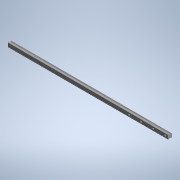
# Autodesk Inventor part: HSR30A128020 Rail(3.5)
Saved by Autodesk Inventor 2022 (Build 260153000, 153)
## iProperties
Category: PARTsolutions
Company: THK
Part Number: HSR30A128020 Rail(3.5)
Material: Generic
Catalog Web Link: www.cadenas.de
Description: Flange Type - Heavy Load HSR-A Rail-
Vendor: THK
Document SubType Name: Modeling
Designer: partserver
Manufacturer: THK
Mass: 162.345 g
Surface Area: 356.21 cm^2
Volume: 162.345 cm^3
Density: 1 g/cm^3
Appearance: PSOLRGB-192-192-192
PSOL_IDENT_0: {$CADENAS_DATA\23d-libs\thk\linear_motion_systems\lm_guide\lm_guide\lm_guide_hsr\four_taped_hole_typ
PSOL_IDENT_1: e\hsr_a\hsr_a_rail.prj},218 {VTYP=3D},{NB=HSR30A128020 Rail},{LINA=HSR30A128020 Rail},{NN=Flange Typ
PSOL_IDENT_2: e - Heavy Load HSR-A Rail},{DATE=08.06.2021 00:57:44},{GEOMDATE=24.12.2019 02:38:17},{VERSION=},{LIN
PSOL_IDENT_3: EID=60},{WBVAR=L,G,GX,TAPH},{WBNUMERIC=L,GX}  {NB=HSR30A128020 Rail},{LINA=HSR30A128020 Rail},{KT=DU
PSOL_IDENT_4: MMY},{MN=HSR30A},{NOB=1},{L=280.0},{G=},{GG='', 'Symmetrical (G1=G2)', 'A', 'Asymmetrical'},{GX=20},
PSOL_IDENT_5: {TAPH=},{GX1=20},{LMIN=98},{LEND=8640.00},{LMING=8.00},{LMAXG=32.00},{W1=28.00},{M1=26.00},{F=80.00}
PSOL_IDENT_6: ,{D1=9.00},{D2=14.00},{HM=12.00},{MAXL=3000.00},{GMIN=8},{GMX=20},{GMAX1=3.3},{G1=20},{G2=20},{NX=1}
PSOL_IDENT_7: ,{H3=7.00},{A=4},{LF=-20},{LM=320},{LL=620},{AA=3},{GMAX=32},{P=4},{PX=0},{VG=3},{VGG=20},{VG1=-1},{
PSOL_IDENT_8: VG2=4},{ND=4.000},{LT=2880},{GA=20.000},{X=0.000},{S1=8.000},{L1=15.000},{NOTE=MIN}
NB: HSR30A128020 Rail
NN: Flange Type - Heavy Load HSR-A Rail
NBSYN: $MN.$NOB.$L.$G.$GX.$TAPH. Rail
LINA: HSR30A128020 Rail
CATALOG: THK
MN: HSR30A
NOB: 1
L: 280
G: Symmetrical (G1=G2)
GX: 20
TAPH: Standard
LEND: 8640
LMING: 8
LMAXG: 32
W1: 28
M1: 26
F: 80
D1: 9
D2: 14
HM: 12
MAXL: 3000
H3: 7
ND: 4
GA: 20
X: 0
S1: 8
L1: 15
NOTE: 0
SUPPLIER: THK
ARTICLENO: HSR30A128020 Rail
BOMINFO: HSR30A128020 Rail
CREATOR: CADENAS GmbH
Title: HSR30A128020 Rail
Author: Cadenas PARTsolutions
Autodesk Inventor part; units mm, degrees
sketch "Sketch_17" plane through (-20, 0, 0) normal (1, 0, 0) x (0, 0, -1)
  line L0 (-14, 1.5) -> (-12.5, 0)
  line L1 (-12.5, 0) -> (-7.75, 0)
  line L2 (-7.75, 0) -> (-7.25, 0.5)
  line L3 (-7.25, 0.5) -> (-3.75, 0.5)
  line L4 (-3.75, 0.5) -> (-3.25, 0)
  line L5 (-3.25, 0) -> (3.25, 0)
  line L6 (3.25, 0) -> (3.75, 0.5)
  line L7 (3.75, 0.5) -> (7.25, 0.5)
  line L8 (7.25, 0.5) -> (7.75, 0)
  line L9 (7.75, 0) -> (12.5, 0)
  line L10 (12.5, 0) -> (14, 1.5)
  line L11 (14, 1.5) -> (14, 6.3)
  line L12 (14, 6.3) -> (9.3003, 10.9996)
  line L13 (9.3003, 10.9996) -> (9.3003, 15.0794)
  line L14 (9.3003, 15.0794) -> (10.9996, 16.7787)
  arc A0 (13.5309, 19.31) -> (10.9996, 16.7787) centre (13.8696, 16.4399) ccw
  line L15 (13.5309, 19.31) -> (14, 19.7791)
  line L16 (14, 19.7791) -> (14, 22.215)
  line L17 (14, 22.215) -> (13.5245, 22.6905)
  arc A1 (11.0003, 25.2147) -> (13.5245, 22.6905) centre (13.8696, 25.5598) ccw
  line L18 (11.0003, 25.2147) -> (10.215, 26)
  line L19 (10.215, 26) -> (-10.215, 26)
  line L20 (-10.215, 26) -> (-11.0003, 25.2147)
  arc A2 (-13.5245, 22.6905) -> (-11.0003, 25.2147) centre (-13.8696, 25.5598) ccw
  line L21 (-13.5245, 22.6905) -> (-14, 22.215)
  line L22 (-14, 22.215) -> (-14, 19.7791)
  line L23 (-14, 19.7791) -> (-13.5309, 19.31)
  arc A3 (-10.9996, 16.7787) -> (-13.5309, 19.31) centre (-13.8696, 16.4399) ccw
  line L24 (-10.9996, 16.7787) -> (-9.3003, 15.0794)
  line L25 (-9.3003, 15.0794) -> (-9.3003, 10.9996)
  line L26 (-9.3003, 10.9996) -> (-14, 6.3)
  line L27 (-14, 6.3) -> (-14, 1.5)
  constraints: 56 end point, 8 point on circle, 4 centre point
extrude "Extrusion1" add sketch "Sketch_17" along normal blind 1066.8
sketch "Sketch2" plane through (-20, 26, 10.215) normal (0, 1, 0) x (1, 0, 0)
  point P0 (20, 10.215)
hole "Hole1" at (0, 26, 0) direction (0, -1, 0) diameter 9 depth 26 counterbore diameter 14 counterbore depth 12
pattern_linear "Rectangular Pattern1" count 4 spacing 80 along (1, 0, 0) of "Hole1"
ref_plane "4dummy_XY" through (0, 0, 0) normal (1, 0, 0) x (0, 0, -1)
ref_plane "4dummy_YZ" through (0, 0, 0) normal (0, 0, -1) x (0, 1, 0)
ref_plane "4dummy_ZX" through (0, 0, 0) normal (0, 1, 0) x (1, 0, 0)
ref_plane "4slide_XY" through (-20, 7, 0) normal (1, 0, 0) x (0, 0, -1)
ref_plane "4slide_YZ" through (-20, 7, 0) normal (0, 0, -1) x (0, 1, 0)
ref_plane "4slide_ZX" through (-20, 7, 0) normal (0, 1, 0) x (1, 0, 0)
ref_plane "4track_XY" through (0, 0, 0) normal (0, 0, 1) x (1, 0, 0)
ref_plane "4track_YZ" through (0, 0, 0) normal (1, 0, 0) x (0, 1, 0)
ref_plane "4track_ZX" through (0, 0, 0) normal (0, 1, 0) x (0, 0, 1)
body "Solid1"
